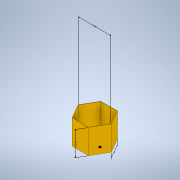
# Autodesk Inventor part: HS-01
Saved by Autodesk Inventor 2022 (Build 260153000, 153)
## iProperties
Company: El Camino College
Created: 2023-05-12
Part Number: HS-01
Material: Aluminum 6061 Painted
Document SubType Name: Modeling
Designer: Edgar Tejada
Density: 2.7 g/cm^3
Appearance: Aluminum - Flat(1)
Mass: 1941.86 g
Surface Area: 4563.41 cm^2
Volume: 719.208 cm^3
Description: Hexagonal Outershell
Author: Edgar Tejada
Title: Hexagonal Shell
Autodesk Inventor part; units mm, degrees
ref_plane "YZ Plane" through (0, 0, 0) normal (1, 0, 0) x (0, 1, 0)
ref_plane "XZ Plane" through (0, 0, 0) normal (0, 1, 0) x (-1, 0, 0)
ref_plane "XY Plane" through (0, 0, 0) normal (0, 0, 1) x (1, 0, 0)
sketch "Sketch1" plane through (0, 0, 0) normal (0, 1, 0) x (-1, 0, 0)
  circle A0 centre (0, 0) radius 95.25 construction
  circle A1 centre (0, 0) radius 120.65 construction
  line L0 (-69.6573, -120.65) -> (-139.3146, 0)
  line L1 (-139.3146, 0) -> (-69.6573, 120.65)
  line L2 (-69.6573, 120.65) -> (69.6573, 120.65)
  line L3 (69.6573, 120.65) -> (139.3146, 0)
  line L4 (139.3146, 0) -> (69.6573, -120.65)
  line L5 (69.6573, -120.65) -> (-69.6573, -120.65)
  line L6 (142.4896, 0) -> (71.2448, 123.3996)
  line L7 (71.2448, 123.3996) -> (-71.2448, 123.3996)
  line L8 (-71.2448, 123.3996) -> (-142.4896, 0)
  line L9 (-142.4896, 0) -> (-71.2448, -123.3996)
  line L10 (-71.2448, -123.3996) -> (71.2448, -123.3996)
  line L11 (71.2448, -123.3996) -> (142.4896, 0)
  dimension "d0" = 190.5
  dimension "d1" = 25.4
  dimension "d2" = 3.175
  constraints: 24 end point, 3 coincident, 2 centre point, 1 horizontal alignment, 1 tangent, 18 other
  measures "d0" diameter of A0
  measures "d1" radial gap between concentric circles of A1 A0
  measures "d2" distance of L3.end L6.start
extrude "Extrusion1" add sketch "Sketch1" along normal blind 209.55 contours L0 L1 L2 L3 L4 L5 | L11 L10 L9 L8 L7 L6
shell "Shell1" thickness 3.175 removed faces 1 at (47.4965, 209.55, 0)
sketch "Sketch2" plane through (142.4896, 0, 0) normal (0.866, 0, 0.5) x (0.5, 0, -0.866)
  circle A0 centre (-71.2448, 50.8) radius 9.525
  line L0 (-142.4896, 0) -> (0, 0) projected
  point P0 (-71.2448, 0)
  point P1 (-71.2448, 0)
  dimension "d15" = 19.05
  dimension "d16" = 50.8
  constraints: 1 centre point, 1 midpoint, 1 vertical alignment
  measures "d15" diameter of A0
  measures "d16" distance from line of L0 A0.centre
extrude "Extrusion2" cut sketch "Sketch2" against normal up to next
sketch "Sketch3" plane through (0, 0, 0) normal (0, -1, 0) x (1, 0, 0)
  line L0 (-71.2448, 123.3996) -> (71.2448, 123.3996) projected
  circle A0 centre (0, 103.232) radius 1.7526
  line L1 (142.4896, 0) -> (71.2448, -123.3996) projected
  line L2 (106.8672, -61.6998) -> (130.6924, -61.6998) construction
  line L3 (-71.2448, -123.3996) -> (-142.4896, 0) projected
  line L4 (-106.8672, -61.6998) -> (-83.042, -61.6998) construction
  circle A1 centre (-89.4016, -51.616) radius 1.7526
  circle A2 centre (89.4016, -51.616) radius 1.7526
  point P0 (0, 0)
  dimension "d20" = 3.5052
  dimension "d21" = 20.1676
  dimension "d26" = 3.5052
  dimension "d27" = 3.5052
  dimension "d28" = 20.1676
  dimension "d29" = 20.1676
  constraints: 4 end point, 3 centre point, 2 horizontal, 2 midpoint
  measures "d20" diameter of A0
  measures "d21" distance from line of L0 A0.centre
  measures "d26" diameter of A1
  measures "d27" diameter of A2
  measures "d28" distance from line of L1 A2.centre
  measures "d29" distance from line of L3 A1.centre
extrude "Extrusion3" cut sketch "Sketch3" against normal blind 12.7
thread "Thread1" size "6-32 UNC" class "2B" standard "ANSI Unified Screw Threads" full length
thread "Thread2" size "6-32 UNC" class "2B" standard "ANSI Unified Screw Threads" full length
thread "Thread3" size "6-32 UNC" class "2B" standard "ANSI Unified Screw Threads" full length
sketch "Sketch4" plane through (71.2448, 0, -123.3996) normal (0, 0, -1) x (-1, 0, 0)
  line L0 (3.2998, 144.145) -> (139.1898, 144.145) construction
  line L1 (139.1898, 144.145) -> (139.1898, 8.255) construction
  line L2 (139.1898, 8.255) -> (3.2998, 8.255) construction
  line L3 (3.2998, 8.255) -> (3.2998, 144.145) construction
  line L4 (3.2998, 144.145) -> (139.1898, 8.255) construction
  line L5 (139.1898, 144.145) -> (3.2998, 8.255) construction
  line L6 (0, 0) -> (142.4896, 0) projected
  circle A0 centre (139.1898, 144.145) radius 1.7996
  circle A1 centre (3.2998, 144.145) radius 1.7996
  circle A2 centre (3.2998, 8.255) radius 1.7996
  circle A3 centre (139.1898, 8.255) radius 1.7996
  point P0 (71.2448, 0)
  point P1 (71.2448, 76.2)
  point P2 (71.2448, 76.2)
  point P3 (71.2448, 0)
  dimension "d38" = 135.89
  dimension "d39" = 76.2
  dimension "d40" = 3.5992
  constraints: 12 end point, 4 centre point, 4 coincident, 4 midpoint, 3 equal radius, 2 parallel, 2 perpendicular, 1 horizontal, 1 vertical alignment
  measures "d38" distance of L0.start L0.end
  measures "d39" distance of point (71.245, 76.2) point (71.245, 0)
  measures "d40" diameter of A0
sketch "Sketch5" plane through (-142.4896, 0, 0) normal (-0.866, 0, -0.5) x (-0.5, 0, 0.866)
  line L0 (-139.1898, 144.145) -> (-3.2998, 144.145) construction
  line L1 (-3.2998, 144.145) -> (-3.2998, 8.255) construction
  line L2 (-3.2998, 8.255) -> (-139.1898, 8.255) construction
  line L3 (-139.1898, 8.255) -> (-139.1898, 144.145) construction
  line L4 (-139.1898, 144.145) -> (-3.2998, 8.255) construction
  line L5 (-3.2998, 144.145) -> (-139.1898, 8.255) construction
  line L6 (0, 0) -> (-142.4896, 0)
  circle A0 centre (-3.2998, 144.145) radius 1.7996
  circle A1 centre (-139.1898, 144.145) radius 1.7996
  circle A2 centre (-139.1898, 8.255) radius 1.7996
  circle A3 centre (-3.2998, 8.255) radius 1.7996
  line L7 (-142.4896, 0) -> (0, 0) projected
  point P0 (-71.2448, 0)
  point P1 (-71.2448, 0)
  point P2 (-71.2448, 76.2)
  point P3 (-71.2448, 76.2)
  point P4 (-71.2448, 0)
  point P5 (-71.2448, 0)
  point P6 (-71.2448, 76.2)
  point P7 (-71.2448, 0)
  dimension "d41" = 135.89
  dimension "d42" = 76.2
  dimension "d43" = 3.5992
  constraints: 14 end point, 9 midpoint, 4 centre point, 4 coincident, 3 equal radius, 3 vertical alignment, 2 parallel, 2 perpendicular, 1 collinear, 1 horizontal
  measures "d41" distance of L0.start L0.end
  measures "d42" distance of point (-71.245, 76.2) point (-71.245, 0)
  measures "d43" diameter of A0
extrude "Extrusion4" cut sketch "Sketch4" against normal up to next
extrude "Extrusion5" cut sketch "Sketch5" against normal up to next
equation "\"d5\" = d2"
body "Solid1"
